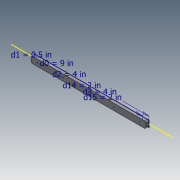
# Autodesk Inventor part: VP BOX LIMIT SPACER
Saved by Autodesk Inventor 2018.3 (Build 223284000, 284)
## iProperties
Created: 2020-02-03
Material: Generic
Vendor: HHMI: JRC - ID&F
Document SubType Name: Modeling
Designer: arnoldj
Density: 1 g/cm^3
Appearance: Default
RuleStatus: InUse
AfterDocSave0: file://Part Number Cleaner
DESIGN DEPARTMENT: HHMI: JRC - ID&F
ALTERED ITEM PART NUMBER: N/A
ALTERED ITEM VENDOR: N/A
ALTERED ITEM DESCRIPTION: N/A
Author: arnoldj
Revision Number: 0
Autodesk Inventor part; units mm, degrees
ref_plane "YZ Plane" through (0, 0, 0) normal (1, 0, 0) x (0, 1, 0)
ref_plane "XZ Plane" through (0, 0, 0) normal (0, 1, 0) x (-1, 0, 0)
ref_plane "XY Plane" through (0, 0, 0) normal (0, 0, 1) x (1, 0, 0)
sketch "Sketch1" plane through (0, 0, 0) normal (0, 0, 1) x (1, 0, 0)
  line L0 (0, 8.89) -> (0, -8.89) projected
  line L1 (-160.02, 0) -> (160.02, 0) projected
  line L2 (114.3, -6.35) -> (-114.3, -6.35)
  line L3 (-114.3, -6.35) -> (-114.3, 6.35)
  line L4 (-114.3, 6.35) -> (114.3, 6.35)
  line L5 (114.3, 6.35) -> (114.3, -6.35)
  line L6 (114.3, -6.35) -> (-114.3, 6.35) construction
  line L7 (-114.3, -6.35) -> (114.3, 6.35) construction
  point P0 (0, 0)
  point P1 (-101.6, 0)
  point P2 (101.6, 0)
  point P3 (0, 0)
  point P4 (-50.8, 0)
  point P5 (50.8, 0)
  dimension "d0" = 228.6
  dimension "d1" = 12.7
  dimension "d2" = 101.6
  dimension "d3" = 101.6
  dimension "d14" = 50.8
  dimension "d15" = 50.8
  constraints: 12 end point, 4 point on line, 2 midpoint, 2 parallel, 1 coincident, 1 horizontal, 1 perpendicular
  measures "d0" distance of L3.end L4.end
  measures "d1" distance of L2.end L3.end
  measures "d2" distance from line of L0 point (-101.6, 0)
  measures "d3" distance from line of L0 point (101.6, 0)
  measures "d14" distance from line of L0 point (-50.8, 0)
  measures "d15" distance from line of L0 point (50.8, 0)
extrude "Extrusion1" add sketch "Sketch1" along normal blind 5.842
hole "Hole1" at (-101.6, 0, 0) at (101.6, 0, 0) at (0, 0, 0) at (50.8, 0, 0) at (-50.8, 0, 0) direction (0, 0, 1) diameter 1.524 end through all
fillet "Fillet1" radius 3.175 4 edges at (114.3, -6.35, 2.921) (114.3, 6.35, 2.921) (-114.3, -6.35, 2.921) (-114.3, 6.35, 2.921)
body "Solid1"
